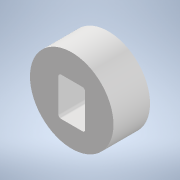
# Autodesk Inventor part: 00_SM05LC-toRMS
Saved by Autodesk Inventor 2022 (Build 260153000, 153)
## iProperties
Created: 2021-10-27
Part Number: 00_SM05LC-toRMS
Material: Generic
Document SubType Name: Modeling
Designer: diederichbenedict
Density: 1 g/cm^3
Appearance: Default
Author: diederichbenedict
Autodesk Inventor part; units mm, degrees
ref_plane "YZ Plane" through (0, 0, 0) normal (1, 0, 0) x (0, 1, 0)
ref_plane "XZ Plane" through (0, 0, 0) normal (0, 1, 0) x (-1, 0, 0)
ref_plane "XY Plane" through (0, 0, 0) normal (0, 0, 1) x (1, 0, 0)
sketch "Sketch1" plane through (0, 0, 0) normal (0, 0, 1) x (1, 0, 0)
  line L0 (0, 0.5) -> (0, 9.6) projected
  arc A0 (0, 9.6) -> (-0.5, 10.1) centre (-0.5, 9.6) ccw projected
  line L1 (-0.5, 10.1) -> (-6.4, 10.1) projected
  arc A1 (-6.4, 10.1) -> (-6.9, 9.6) centre (-6.4, 9.6) ccw projected
  line L2 (-6.9, 9.6) -> (-6.9, 0.5) projected
  arc A2 (-6.9, 0.5) -> (-6.4, 0) centre (-6.4, 0.5) ccw projected
  line L3 (-6.4, 0) -> (-0.5, 0) projected
  arc A3 (-0.5, 0) -> (0, 0.5) centre (-0.5, 0.5) ccw projected
  line L4 (-2.6, 8.25) -> (-2.6, 8.8) projected
  line L5 (-1.15, 8.25) -> (-2.6, 8.25) projected
  line L6 (-1.15, 3.65) -> (-1.15, 8.25) projected
  line L7 (-1.8, 3.65) -> (-1.15, 3.65) projected
  line L8 (-1.8, 2.85) -> (-1.8, 3.65) projected
  line L9 (-1.15, 2.85) -> (-1.8, 2.85) projected
  line L10 (-1.15, 1.75) -> (-1.15, 2.85) projected
  line L11 (-2.15, 1.75) -> (-1.15, 1.75) projected
  line L12 (-2.15, 0.75) -> (-2.15, 1.75) projected
  line L13 (-4.75, 0.75) -> (-2.15, 0.75) projected
  line L14 (-4.75, 1.75) -> (-4.75, 0.75) projected
  line L15 (-5.75, 1.75) -> (-4.75, 1.75) projected
  line L16 (-5.75, 2.85) -> (-5.75, 1.75) projected
  line L17 (-5.1, 2.85) -> (-5.75, 2.85) projected
  line L18 (-5.1, 3.65) -> (-5.1, 2.85) projected
  line L19 (-5.75, 3.65) -> (-5.1, 3.65) projected
  line L20 (-5.75, 8.25) -> (-5.75, 3.65) projected
  line L21 (-4.3, 8.25) -> (-5.75, 8.25) projected
  line L22 (-4.3, 8.8) -> (-4.3, 8.25) projected
  line L23 (-2.6, 8.8) -> (-4.3, 8.8) projected
  circle A4 centre (-3.45, 5.6) radius 0.9 projected
  circle A5 centre (-3.45, 5.6) radius 11.4128
  line L24 (-7.1, 0.5) -> (-7.1, 9.6)
  arc A6 (-6.4, 10.3) -> (-7.1, 9.6) centre (-6.4, 9.6) ccw
  line L25 (-6.4, 10.3) -> (-0.5, 10.3)
  arc A7 (0.2, 9.6) -> (-0.5, 10.3) centre (-0.5, 9.6) ccw
  line L26 (0.2, 9.6) -> (0.2, 0.5)
  arc A8 (-0.5, -0.2) -> (0.2, 0.5) centre (-0.5, 0.5) ccw
  line L27 (-0.5, -0.2) -> (-6.4, -0.2)
  arc A9 (-7.1, 0.5) -> (-6.4, -0.2) centre (-6.4, 0.5) ccw
  point P0 (0, 0)
  dimension "d0" = 0.2
  constraints: 8 end point, 8 point on circle, 5 centre point, 1 coincident, 7 other
  measures "d0" distance between parallel lines of L2 L24
extrude "Extrusion1" add sketch "Sketch1" against normal blind 10 contours A5
body "Solid1"
